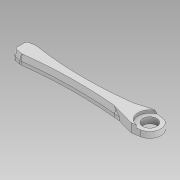
# Autodesk Inventor part: PocketPointBar2
Saved by Autodesk Inventor 2021 (Build 250183000, 183)
## iProperties
Created: 2021-02-18
Part Number: PocketPointBar2
Material: 一般
Document SubType Name: Modeling
Designer: kumagai
Density: 1 g/cm^3
Appearance: 既定
Author: kumagai
Autodesk Inventor part; units mm, degrees
ref_plane "YZ Plane" through (0, 0, 0) normal (1, 0, 0) x (0, 1, 0)
ref_plane "XZ Plane" through (0, 0, 0) normal (0, 1, 0) x (-1, 0, 0)
ref_plane "XY Plane" through (0, 0, 0) normal (0, 0, 1) x (1, 0, 0)
sketch "スケッチ1" plane through (0, 0, 0) normal (0, 1, 0) x (-1, 0, 0)
  line L0 (0, -183.504) -> (0, 210.204) projected
  line L1 (-14.3452, 0) -> (57.8075, 0) projected
  arc A0 (-0.6536, 3.9462) -> (-0.5779, -3.958) centre (0, 0) ccw
  arc A1 (44.1796, -3.0855) -> (10.2032, -2.4465) centre (24.85, -127.26) ccw
  line L2 (47.5, 2.5) -> (47.5, -2.5)
  line L3 (-0.5779, -3.958) -> (2.4697, -4.403)
  circle A2 centre (0, 0) radius 2.55
  line L4 (47.5, 2.5) -> (44.0175, 3.1141)
  line L5 (2.4697, -4.403) -> (8.2169, -2.6796)
  line L6 (8.2169, -2.6796) -> (10.2032, -2.4465)
  arc A3 (10.1741, 2.6446) -> (44.0175, 3.1141) centre (25, 153.96) ccw
  line L7 (10.1741, 2.6446) -> (8.1836, 2.8396)
  line L8 (8.1836, 2.8396) -> (2.4045, 4.4527)
  line L9 (2.4045, 4.4527) -> (-0.6536, 3.9462)
  line L10 (47.5, -2.5) -> (44.1796, -3.0855)
  point P0 (0, 4)
  dimension "d1" = 8
  dimension "d5" = 5.1
  dimension "d13" = 2.5
  dimension "d16" = 47.5
  dimension "d17" = 22.65
  dimension "d23" = 25
  dimension "d24" = 2
  dimension "d25" = 10
  dimension "d26" = 6
  dimension "d29" = 22.5
  dimension "d30" = 153.96
  dimension "d31" = 152.04
  dimension "d32" = 127.26
  dimension "d33" = 125.67
  dimension "d34" = 2
  dimension "d35" = 6
  dimension "d36" = 10
  dimension "d37" = 25
  dimension "d38" = 2.5
  dimension "d41" = 10
  dimension "d42" = 10
  constraints: 18 end point, 6 point on circle, 4 centre point, 4 tangent, 2 coincident, 1 point on line, 1 vertical
  measures "d1" diameter of A0
  measures "d5" diameter of A2
  measures "d13" distance from line of L1 L2.start
  measures "d16" distance between parallel lines of L2 L0
  measures "d17" distance from line of A1.centre L2
  measures "d23" angle of L3 L5
  measures "d24" distance of L5.end L6.end
  measures "d25" angle of L5 L6
  measures "d26" distance of L3.end L5.end
  measures "d29" distance from line of L2 A3.centre
  measures "d30" distance from line of A3.centre L1
  measures "d31" radius of A3
  measures "d32" distance from line of A1.centre L1
  measures "d33" radius of A1
  measures "d34" distance of L7.start L7.end
  measures "d35" distance of L7.end L8.end
  measures "d36" angle of L8 L7
  measures "d37" angle of L9 L8
  measures "d38" distance from line of L2.end L1
  measures "d41" angle of L1 L10
  measures "d42" angle of L4 L1
extrude "押し出し1" add sketch "スケッチ1" along normal blind 3.2 contours L3 A0 L1 A2 L0 | L0 A2 L1 L2 L10 A1 L6 L5 L3 | L1 A0 L9 L0 A2 | A2 L0 L9 L8 L7 A3 L4 L2 L1
fillet "フィレット1" radius 1.5 6 edges at (-47.5, 1.6, 2.5) (-44.0175, 1.6, 3.1141) (-47.5, 1.6, -2.5) (-44.1796, 1.6, -3.0855) (-2.4697, 1.6, -4.403) (-8.2169, 1.6, -2.6796)
sketch "スケッチ2" plane through (0, 3.2, 0) normal (0, 1, 0) x (1, 0, 0)
  circle A0 centre (0, 0) radius 4.25
  dimension "d9" = 8.5
  constraints: 1 centre point, 1 coincident
  measures "d9" diameter of A0
extrude "押し出し2" cut sketch "スケッチ2" against normal blind 1
chamfer "面取り1" distance 0.5 distance2 2 8 edges at (-44.0176, 3.2, 3.0971) (-45.2503, 3.2, 2.8967) (-47.1491, 3.2, 2.2055) (-47.5, 3.2, 0) (-47.1491, 3.2, -2.2055) (-44.1802, 3.2, -3.0651) (-27.0898, 3.2, -1.61) (-1.4919, 3.2, -4.2602) measured on face at (-46.766, 3.2, -1.8841) measured on face at (-45.1635, 3.2, 2.4043) measured on face at (-46.766, 3.2, 1.8841) measured on face at (-44.005, 3.2, 2.5973) measured on face at (-1.5064, 3.2, -4.1613) measured on face at (-47, 3.2, 0) measured on face at (-44.1746, 3.2, -2.5651) measured on face at (-27.0987, 3.2, -1.11)
